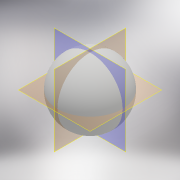
# Autodesk Inventor part: 零件2
Saved by Autodesk Inventor 2017 (Build 210142000, 142)
## iProperties
Part Number: 零件2
Material: 一般
Document SubType Name: Modeling
Designer: 吳宜賢
Density: 1 g/cm^3
Appearance: 預設
Author: 吳宜賢
Autodesk Inventor part; units mm, degrees
sketch "草圖1" plane through (0, 0, 0) normal (1, 0, 0) x (0, 1, 0)
  line L0 (0, 3.6) -> (0, -0.6) projected
  line L1 (-4.2, 0) -> (4.2, 0) projected
  arc A0 (3, 0) -> (-3, 0) centre (0, 0) ccw
  line L2 (-3, 0) -> (3, 0)
  dimension "d0" = 6
  constraints: 2 end point, 2 point on circle, 2 point on line, 1 centre point, 1 coincident
  measures "d0" diameter of A0
revolve "迴轉1" add sketch "草圖1" angle 360 about axis through (0, -3, 0) along (0, 1, 0)
